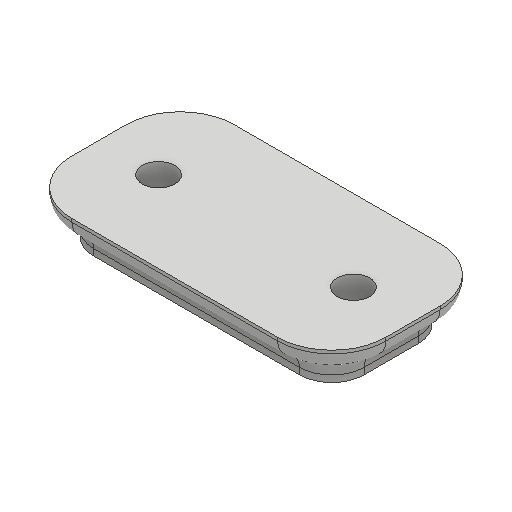
# Autodesk Inventor part: 3DP_ABS_Y_Axis_Belt_Mount_Spacer
Saved by Autodesk Inventor 2026.1 (Build 301233000, 233)
## iProperties
Created: 2017-05-25
Part Number: 3DP_ABS_Y_Axis_Belt_Mount_Spacer
Material: Ogólny
Document SubType Name: Modeling
Designer: Andrzej
Density: 1 g/cm^3
Appearance: Domyślna
Author: Andrzej
Autodesk Inventor part; units mm, degrees
ref_plane "YZ Plane" through (0, 0, 0) normal (1, 0, 0) x (0, 1, 0)
ref_plane "XZ Plane" through (0, 0, 0) normal (0, 1, 0) x (-1, 0, 0)
ref_plane "XY Plane" through (0, 0, 0) normal (0, 0, 1) x (1, 0, 0)
sketch "Szkic1" plane through (0, 0, 0) normal (0, 0, 1) x (1, 0, 0)
  line L0 (-17.1731, 6.2025) -> (7.8269, 6.2025)
  line L1 (7.8269, 6.2025) -> (7.8269, -4.7975)
  line L2 (7.8269, -4.7975) -> (-17.1731, -4.7975)
  line L3 (-17.1731, -4.7975) -> (-17.1731, 6.2025)
  point P0 (0, 0)
  point P1 (-13.6731, 0.7025)
  point P2 (4.3269, 0.7025)
  dimension "d0" = 25
  dimension "d1" = 11
  dimension "d2" = 5.5
  dimension "d3" = 5.5
  dimension "d4" = 3.5
  dimension "d5" = 3.5
  constraints: 8 end point, 2 parallel, 1 horizontal, 1 perpendicular
  measures "d0" distance of L1.end L2.end
  measures "d1" distance of L0.end L1.end
  measures "d2" distance from line of L0 point (-13.673, 0.703)
  measures "d3" distance from line of L0 point (4.327, 0.703)
  measures "d4" distance from line of L3 point (-13.673, 0.703)
  measures "d5" distance from line of L1 point (4.327, 0.703)
extrude "Wyciągnięcie proste1" add sketch "Szkic1" along normal blind 2
hole "Otwór1" at (-13.6731, 0.7025, 0) at (4.3269, 0.7025, 0) direction (0, 0, 1) diameter 3 end through all
fillet "Zaokrąglenie1" radius 3 4 edges at (-17.1731, 6.2025, 1) (-17.1731, -4.7975, 1) (7.8269, 6.2025, 1) (7.8269, -4.7975, 1)
sketch "Szkic3" plane through (0, 0, 2) normal (0, 0, 1) x (1, 0, 0)
  arc A0 (4.8269, -4.7975) -> (7.8269, -1.7975) centre (4.8269, -1.7975) ccw projected
  line L0 (7.8269, -1.7975) -> (7.8269, 3.2025) projected
  arc A1 (7.8269, 3.2025) -> (4.8269, 6.2025) centre (4.8269, 3.2025) ccw projected
  line L1 (4.8269, 6.2025) -> (-14.1731, 6.2025) projected
  arc A2 (-14.1731, 6.2025) -> (-17.1731, 3.2025) centre (-14.1731, 3.2025) ccw projected
  line L2 (-17.1731, 3.2025) -> (-17.1731, -1.7975) projected
  arc A3 (-17.1731, -1.7975) -> (-14.1731, -4.7975) centre (-14.1731, -1.7975) ccw projected
  line L3 (-14.1731, -4.7975) -> (4.8269, -4.7975) projected
  circle A4 centre (-13.6731, 0.7025) radius 1.5 projected
  circle A5 centre (4.3269, 0.7025) radius 1.5 projected
  line L4 (-14.1731, 8.2025) -> (4.8269, 8.2025)
  arc A6 (9.8269, 3.2025) -> (4.8269, 8.2025) centre (4.8269, 3.2025) ccw
  line L5 (9.8269, 3.2025) -> (9.8269, -1.7975)
  arc A7 (4.8269, -6.7975) -> (9.8269, -1.7975) centre (4.8269, -1.7975) ccw
  line L6 (4.8269, -6.7975) -> (-14.1731, -6.7975)
  arc A8 (-19.1731, -1.7975) -> (-14.1731, -6.7975) centre (-14.1731, -1.7975) ccw
  line L7 (-19.1731, -1.7975) -> (-19.1731, 3.2025)
  arc A9 (-14.1731, 8.2025) -> (-19.1731, 3.2025) centre (-14.1731, 3.2025) ccw
  point P0 (0, 0)
  dimension "d16" = 2
  constraints: 8 end point, 8 point on circle, 4 centre point, 7 other
  measures "d16" distance between parallel lines of L1 L4
extrude "Wyciągnięcie proste2" add sketch "Szkic3" along normal blind 2 contours L3 A3 L2 A2 L1 A1 L0 A0 | L4 A6 L5 A7 L6 A8 L7 A9
fillet "Zaokrąglenie2" radius 1.7 16 edges at (8.3624, -5.333, 2) (-4.6731, -6.7975, 2) (-17.7087, -5.333, 2) (-19.1731, 0.7025, 2) (-17.7087, 6.7381, 2) (-4.6731, 8.2025, 2) (8.3624, 6.7381, 2) (9.8269, 0.7025, 2) (6.9482, 5.3238, 2) (-4.6731, 6.2025, 2) (-16.2944, 5.3238, 2) (-17.1731, 0.7025, 2) (-16.2944, -3.9188, 2) (-4.6731, -4.7975, 2) (6.9482, -3.9188, 2) (7.8269, 0.7025, 2)
equation "\"d5\" = d4"
